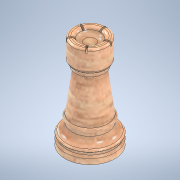
# Autodesk Inventor part: wieża
Saved by Autodesk Inventor 2021 (Build 250183000, 183)
## iProperties
Created: 2021-01-07
Part Number: wieża
Material: Drewno (brzoza)
Document SubType Name: Modeling
Designer: Adam
Density: 0.55 g/cm^3
Appearance: Brzoza — naturalna — polerowana
Author: Adam
Autodesk Inventor part; units mm, degrees
ref_plane "YZ Plane" through (0, 0, 0) normal (1, 0, 0) x (0, 1, 0)
ref_plane "XZ Plane" through (0, 0, 0) normal (0, 1, 0) x (-1, 0, 0)
ref_plane "XY Plane" through (0, 0, 0) normal (0, 0, 1) x (1, 0, 0)
sketch "Szkic1" plane through (0, 0, 0) normal (1, 0, 0) x (0, 1, 0)
  line L0 (0, 10) -> (0, -4)
  line L1 (0, 10) -> (53, 10)
  line L2 (0, -4) -> (4, -4)
  line L3 (4, -4) -> (4, -3)
  line L4 (4, -3) -> (5, -3)
  line L5 (5, -3) -> (5, -4)
  line L6 (5, -4) -> (7, -4)
  line L7 (11, 0) -> (13, 0)
  arc A0 (11, 0) -> (7, -4) centre (11, -4) ccw
  line L8 (13, 0) -> (13, -1)
  line L9 (13, -1) -> (15, -1)
  line L10 (15, -1) -> (15, 0)
  line L11 (38, 3) -> (15, 0)
  line L12 (38, 3) -> (38, 2)
  line L13 (38, 2) -> (40, 2)
  line L14 (40, 2) -> (40, 1)
  line L15 (40, 1) -> (42, 1)
  line L16 (42, 1) -> (42, 0.5)
  line L17 (42, 0.5) -> (53, 0.5)
  line L18 (53, 0.5) -> (53, 10)
  point P0 (0, 0)
  constraints: 38 end point, 10 perpendicular, 5 vertical, 3 horizontal, 2 point on circle, 1 centre point, 1 point on line, 1 tangent
revolve "Obrót1" add sketch "Szkic1" angle 360 about axis through (0, 0, 10) along (0, 1, 0)
fillet "Zaokrąglenie1" radius 1 1 edges at (0, 4, 24)
fillet "Zaokrąglenie2" radius 1 2 edges at (0, 5, 24) (0, 7, 24)
fillet "Zaokrąglenie4" radius 1 1 edges at (0, 15, 21)
fillet "Zaokrąglenie5" radius 1 1 edges at (0, 13, 21)
fillet "Zaokrąglenie6" radius 1 2 edges at (0, 40, 19) (0, 42, 19)
fillet "Zaokrąglenie7" radius 0.5 1 edges at (0, 38, 18)
fillet "Zaokrąglenie8" radius 1 1 edges at (0, 53, 19.5)
sketch "Szkic2" plane through (0, 53, 10) normal (0, 1, 0) x (1, 0, 0)
  circle A0 centre (0, 0) radius 6
  point P0 (0, 10)
  constraints: 1 centre point
extrude "Wyciągnięcie proste1" cut sketch "Szkic2" against normal blind 3
fillet "Zaokrąglenie9" radius 3 1 edges at (-6, 50, 10)
fillet "Zaokrąglenie10" radius 2 2 edges at (-6, 52.9999, 10) (-6, 53, 10)
sketch "Szkic3" plane through (0, 53, 10) normal (0, 1, 0) x (1, 0, 0)
  circle A0 centre (0, 0) radius 8.5 projected
  circle A1 centre (0, 0) radius 7.5826 projected
  line L0 (-0.0003, 7.5826) -> (-0.0003, 7.5826)
  circle A2 centre (0, 0) radius 5.7495 projected
  line L1 (0.4588, 5.7312) -> (0, 5.7312)
  line L2 (0.4588, 5.7312) -> (-0.4588, 5.7312)
  line L3 (-0.4588, 5.7312) -> (-0.4588, 8.4876)
  line L4 (0.4588, 5.7312) -> (0.4588, 8.4876)
  line L5 (-0.4588, 8.4876) -> (-0.4588, 10)
  line L6 (0.4588, 8.4876) -> (0.4588, 9.9895)
  circle A3 centre (0, 0) radius 10 projected
  arc A4 (-0.4588, 10) -> (0.4588, 9.9895) centre (0.4588, 49.9737) ccw
  line L7 (5.5925, 1.3347) -> (5.3089, 2.2073)
  line L8 (5.3089, 2.2073) -> (7.9304, 3.0591)
  line L9 (7.9304, 3.0591) -> (9.3688, 3.5265)
  arc A5 (9.3688, 3.5265) -> (9.6423, 2.6506) centre (47.6696, 15.0064) ccw
  line L10 (8.214, 2.1865) -> (9.6423, 2.6506)
  line L11 (5.5925, 1.3347) -> (8.214, 2.1865)
  line L12 (2.9976, -4.9063) -> (3.7399, -4.367)
  line L13 (3.7399, -4.367) -> (5.36, -6.597)
  line L14 (5.36, -6.597) -> (6.249, -7.8205)
  arc A6 (6.249, -7.8205) -> (5.5005, -8.3513) centre (29.0027, -40.6992) ccw
  line L15 (4.6178, -7.1363) -> (5.5005, -8.3513)
  line L16 (2.9976, -4.9063) -> (4.6178, -7.1363)
  line L17 (-3.7399, -4.367) -> (-2.9976, -4.9063)
  line L18 (-2.9976, -4.9063) -> (-4.6178, -7.1363)
  line L19 (-4.6178, -7.1363) -> (-5.5067, -8.3598)
  arc A7 (-5.5067, -8.3598) -> (-6.2428, -7.812) centre (-29.7449, -40.1599) ccw
  line L20 (-5.36, -6.597) -> (-6.2428, -7.812)
  line L21 (-3.7399, -4.367) -> (-5.36, -6.597)
  line L22 (-5.3089, 2.2073) -> (-5.5925, 1.3347)
  line L23 (-5.5925, 1.3347) -> (-8.214, 2.1865)
  line L24 (-8.214, 2.1865) -> (-9.6523, 2.6539)
  arc A8 (-9.6523, 2.6539) -> (-9.3588, 3.5232) centre (-47.386, 15.879) ccw
  line L25 (-7.9304, 3.0591) -> (-9.3588, 3.5232)
  line L26 (-5.3089, 2.2073) -> (-7.9304, 3.0591)
  point P0 (0, 10)
  dimension "d23" = 360
  constraints: 54 end point, 17 point on circle, 6 point on line, 5 centre point, 2 coincident, 2 vertical, 1 perpendicular, 74 other
extrude "Wyciągnięcie proste2" cut sketch "Szkic3" against normal blind 2 contours L11 A1 L8 A0 | A0 L9 A3 A5 L10 | L14 A3 A6 L15 A0 | A0 L16 A1 L13 | L11 A2 L8 A1 | A1 L16 A2 L13 | L14 A6 A3 | L4 A1 L3 A0 | A0 L5 A3 A4 L6 | L9 A5 A3 | L7 A2 | L19 A3 A7 L20 A0 | A0 L21 A1 L18 | A2 L12 | L4 A2 L3 A1 | A1 L21 A2 L18 | L19 A7 A3 | L26 A1 L23 A0 | A0 L24 A3 A8 L25 | L5 A4 A3 | L1 L2 A2 | A2 L17 | L26 A2 L23 A1 | L24 A8 A3 | L22 A2
